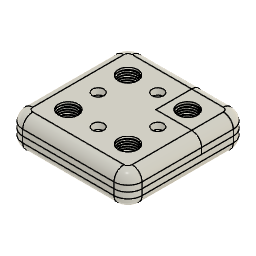
PTFE Mount (Autodesk Fusion 360 design; units mm, degrees)
Autodesk Fusion 360 part; units mm, degrees
sketch "Sketch1" plane through (0, 0, 0) normal (0, 0, 1) x (1, 0, 0)
  line L0 (-30, 0) -> (-30, 30)
  line L1 (-30, 30) -> (0, 30)
  line L2 (-30, 30) -> (30, 30)
  line L3 (30, 30) -> (30, -30)
  line L4 (30, -30) -> (-30, -30)
  line L5 (-30, -30) -> (-30, 30)
  line L6 (-20, 30) -> (-15, 30)
  line L7 (-30, 15) -> (-30, 20)
  point P0 (-15, 15)
  point P1 (15, 15)
  point P2 (15, -15)
  point P3 (-15, -15)
  point P4 (-30, 20)
  point P5 (-20, 30)
  dimension "d1" = 30
  dimension "d2" = 30
  dimension "d3" = 60
  dimension "d4" = 60
  constraint vertical L0
  constraint horizontal L1
  constraint horizontal L2
  constraint vertical L3
  constraint horizontal L4
  constraint vertical L5
  constraint horizontal L6
  constraint vertical L7
  constraint coincident P4 L7.end
  constraint coincident P5 L6.start
  measures "d1" distance of origin L0.start
  measures "d2" distance of origin L1.end
  measures "d3" distance of L0.end L2.end
  measures "d4" distance of L0.end L4.end
extrude "Extrude1" add sketch "Sketch1" along normal blind 8 makes body 1
sketch "Sketch2" plane through (0, 0, 8) normal (0, 0, 1) x (-1, 0, 0)
  line L0 (30, -30) -> (30, 30)
  line L1 (30, 30) -> (-30, 30)
  line L2 (-30, 30) -> (-30, -30)
  line L3 (-30, -30) -> (30, -30)
  circle A0 centre (15, -15) radius 2.075
  point P0 (15, -15)
cylinder "CylinderPrimitive1" cut diameter 4.25 height -14 placed x (1, 0, 0) y (0, 1, 0) z (0, 0, 1) at (-15, 15, 8) bodies 1
cylinder "CylinderPrimitive2" cut diameter 4.25 height -26 placed x (1, 0, 0) y (0, 1, 0) z (0, 0, 1) at (15, 15, 8) bodies 1
cylinder "CylinderPrimitive3" cut diameter 4.25 height -29 placed x (1, 0, 0) y (0, 1, 0) z (0, 0, 1) at (-15, -15, 8) bodies 1
cylinder "CylinderPrimitive4" cut diameter 4.25 height -23 placed x (1, 0, 0) y (0, 1, 0) z (0, 0, 1) at (15, -15, 8) bodies 1
sketch "Sketch10" plane through (0, 0, 8) normal (0, 0, 1) x (-1, 0, 0)
  point P0 (-15, -15)
  point P1 (-15, -15)
  point P2 (-15, 15)
  point P3 (-15, 15)
  point P4 (15, 15)
  point P5 (15, 15)
  constraint coincident P0 P1
  constraint coincident P2 P3
  constraint coincident P4 P5
hole "Hole1" at (-15, 15, 8) at (15, 15, 8) at (15, -15, 8) at (-15, -15, 8) direction (0, 0, -1) diameter 8.526 depth 6.5 tip angle 180 counterbore diameter 9.75 counterbore depth 1 bodies 1
thread "Thread1" "ISO Metric profile 10.0 M10x1.12 6H" major diameter 10.1608 minor diameter 8.9126 pitch 1.12 angle 60 modelled right hand crest width 0.306 on face at (-14.7875, 10.7423, 5.1667) crest through (-10.5437, 15, 6.72) on face at (15.2125, 10.7423, 5.1667) crest through (19.4563, 15, 6.72) on face at (15.2125, -19.2577, 5.1667) crest through (19.4563, -15, 6.72) on face at (-14.7875, -19.2577, 5.1667) crest through (-10.5437, -15, 6.72) on bodies 1
fillet "Fillet1" chord length 10 1 edges at (-30, -30, 4) on bodies 1
fillet "Fillet2" chord length 10 3 edges at (30, -30, 4) (30, 30, 4) (-30, 30, 4) on bodies 1
fillet "Fillet3" radius 5 8 edges at (27.9294, -27.9285, 8) (30, 0, 8) (27.9285, 27.9294, 8) (0, 30, 8) (-27.9294, 27.9285, 8) (-30, 0, 8) (-27.9285, -27.9294, 8) (0, -30, 8) on bodies 1
copy_body "CopyPasteBodies1" bodies 1 makes body 2
move_body "Move1" bodies 2 to x (-1, 0, 0) y (0, 1, 0) z (0, 0, -1) at (0, 0, 0)
sketch "Sketch11" plane through (0, 0, 8) normal (0, 0, 1) x (-1, 0, 0)
  circle A0 centre (15, 15) radius 4.875
  circle A1 centre (-15, -15) radius 4.875
  circle A2 centre (15, -15) radius 4.875
  circle A3 centre (-15, 15) radius 4.875
  spline S0 degree 3 poles (-25, 22.9289) (-25, 23.0652) (-24.9865, 23.2015) (-24.917, 23.549) (-24.8402, 23.756) (-24.5939, 24.1929) (-24.4033, 24.4108) (-23.9063, 24.7861) (-23.5846, 24.9225) (-23.1435, 24.9917) (-23.0362, 25) (-22.9289, 25) knots 0 0 0 0 0.040888 0.040888 0.106308 0.106308 0.191354 0.191354 0.293128 0.293128 0.325306 0.325306 0.325306 0.325306
  line L0 (-25, 22.9289) -> (-25, -22.9289)
  spline S1 degree 3 poles (-22.9289, -25) (-23.0652, -25) (-23.2015, -24.9865) (-23.549, -24.917) (-23.756, -24.8402) (-24.1929, -24.5939) (-24.4108, -24.4033) (-24.7861, -23.9063) (-24.9225, -23.5846) (-24.9917, -23.1435) (-25, -23.0362) (-25, -22.9289) knots 0 0 0 0 0.040888 0.040888 0.106308 0.106308 0.191354 0.191354 0.293128 0.293128 0.325306 0.325306 0.325306 0.325306
  line L1 (-22.9289, -25) -> (22.9289, -25)
  spline S2 degree 3 poles (25, -22.9289) (25, -23.0652) (24.9865, -23.2015) (24.917, -23.549) (24.8402, -23.756) (24.5939, -24.1929) (24.4033, -24.4108) (23.9063, -24.7861) (23.5846, -24.9225) (23.1435, -24.9917) (23.0362, -25) (22.9289, -25) knots 0 0 0 0 0.040888 0.040888 0.106308 0.106308 0.191354 0.191354 0.293128 0.293128 0.325306 0.325306 0.325306 0.325306
  line L2 (25, -22.9289) -> (25, 22.9289)
  spline S3 degree 3 poles (22.9289, 25) (23.0652, 25) (23.2015, 24.9865) (23.549, 24.917) (23.756, 24.8402) (24.1929, 24.5939) (24.4108, 24.4033) (24.7861, 23.9063) (24.9225, 23.5846) (24.9917, 23.1435) (25, 23.0362) (25, 22.9289) knots 0 0 0 0 0.040888 0.040888 0.106308 0.106308 0.191354 0.191354 0.293128 0.293128 0.325306 0.325306 0.325306 0.325306
  line L3 (22.9289, 25) -> (-22.9289, 25)
  point P0 (15, 0)
  point P1 (0, -15)
  point P2 (-15, 0)
  point P3 (0, 15)
  dimension "d31" = 15
  dimension "d32" = 15
  dimension "d33" = 15
  dimension "d34" = 15
  measures "d31" distance of origin P0
  measures "d32" distance of origin P2
  measures "d33" distance of origin P1
  measures "d34" distance of origin P3
hole "Hole2" at (0, 15, 8) at (-15, 0, 8) at (15, 0, 8) at (0, -15, 8) direction (0, 0, -1) diameter 3.2 depth 16 tip angle 180 counterbore diameter 5.75 counterbore depth 3.2 bodies 1
sketch "Sketch12" plane through (0, 0, -8) normal (0, 0, -1) x (1, 0, 0)
  circle A0 centre (15, 15) radius 4.875
  circle A1 centre (-15, -15) radius 4.875
  circle A2 centre (15, -15) radius 4.875
  circle A3 centre (-15, 15) radius 4.875
  spline S0 degree 3 poles (-25, 22.9289) (-25, 23.0652) (-24.9865, 23.2015) (-24.917, 23.549) (-24.8402, 23.756) (-24.5939, 24.1929) (-24.4033, 24.4108) (-23.9063, 24.7861) (-23.5846, 24.9225) (-23.1435, 24.9917) (-23.0362, 25) (-22.9289, 25) knots 0 0 0 0 0.040888 0.040888 0.106308 0.106308 0.191354 0.191354 0.293128 0.293128 0.325306 0.325306 0.325306 0.325306
  line L0 (-25, 22.9289) -> (-25, -22.9289)
  spline S1 degree 3 poles (-22.9289, -25) (-23.0652, -25) (-23.2015, -24.9865) (-23.549, -24.917) (-23.756, -24.8402) (-24.1929, -24.5939) (-24.4108, -24.4033) (-24.7861, -23.9063) (-24.9225, -23.5846) (-24.9917, -23.1435) (-25, -23.0362) (-25, -22.9289) knots 0 0 0 0 0.040888 0.040888 0.106308 0.106308 0.191354 0.191354 0.293128 0.293128 0.325306 0.325306 0.325306 0.325306
  line L1 (-22.9289, -25) -> (22.9289, -25)
  spline S2 degree 3 poles (25, -22.9289) (25, -23.0652) (24.9865, -23.2015) (24.917, -23.549) (24.8402, -23.756) (24.5939, -24.1929) (24.4033, -24.4108) (23.9063, -24.7861) (23.5846, -24.9225) (23.1435, -24.9917) (23.0362, -25) (22.9289, -25) knots 0 0 0 0 0.040888 0.040888 0.106308 0.106308 0.191354 0.191354 0.293128 0.293128 0.325306 0.325306 0.325306 0.325306
  line L2 (25, -22.9289) -> (25, 22.9289)
  spline S3 degree 3 poles (22.9289, 25) (23.0652, 25) (23.2015, 24.9865) (23.549, 24.917) (23.756, 24.8402) (24.1929, 24.5939) (24.4108, 24.4033) (24.7861, 23.9063) (24.9225, 23.5846) (24.9917, 23.1435) (25, 23.0362) (25, 22.9289) knots 0 0 0 0 0.040888 0.040888 0.106308 0.106308 0.191354 0.191354 0.293128 0.293128 0.325306 0.325306 0.325306 0.325306
  line L3 (22.9289, 25) -> (-22.9289, 25)
  line L4 (-17.9055, 1.6058) -> (-17.8435, -1.7134)
  line L5 (-17.8435, -1.7134) -> (-14.9379, -3.3192)
  line L6 (-14.9379, -3.3192) -> (-12.0945, -1.6058)
  line L7 (-12.0945, -1.6058) -> (-12.1565, 1.7134)
  line L8 (-12.1565, 1.7134) -> (-15.0621, 3.3192)
  line L9 (-15.0621, 3.3192) -> (-17.9055, 1.6058)
  line L10 (12.1483, 1.6996) -> (12.1023, -1.6199)
  line L11 (12.1023, -1.6199) -> (14.954, -3.3194)
  line L12 (14.954, -3.3194) -> (17.8517, -1.6996)
  line L13 (17.8517, -1.6996) -> (17.8977, 1.6199)
  line L14 (17.8977, 1.6199) -> (15.046, 3.3194)
  line L15 (15.046, 3.3194) -> (12.1483, 1.6996)
  line L16 (-1.6599, 17.875) -> (-3.3198, 15)
  line L17 (-3.3198, 15) -> (-1.6599, 12.125)
  line L18 (-1.6599, 12.125) -> (1.6599, 12.125)
  line L19 (1.6599, 12.125) -> (3.3198, 15)
  line L20 (3.3198, 15) -> (1.6599, 17.875)
  line L21 (1.6599, 17.875) -> (-1.6599, 17.875)
  line L22 (-1.6599, -12.125) -> (-3.3198, -15)
  line L23 (-3.3198, -15) -> (-1.6599, -17.875)
  line L24 (-1.6599, -17.875) -> (1.6599, -17.875)
  line L25 (1.6599, -17.875) -> (3.3198, -15)
  line L26 (3.3198, -15) -> (1.6599, -12.125)
  line L27 (1.6599, -12.125) -> (-1.6599, -12.125)
  point P0 (0, -15)
  point P1 (0, -15)
  point P2 (-15, 0)
  point P3 (-15, 0)
  point P4 (0, 15)
  point P5 (0, 15)
  point P6 (15, 0)
  point P7 (15, 0)
  point P8 (-15, 0)
  point P9 (15, 0)
  point P10 (0, 15)
  point P11 (0, -15)
  dimension "d40" = 2.875
  dimension "d41" = 2.875
  dimension "d42" = 2.875
  dimension "d43" = 2.875
  constraint coincident P11 P1
  constraint coincident P8 P3
  constraint coincident P10 P5
  constraint coincident P9 P7
  measures "d40" distance of P8 L9
  measures "d41" distance of P9 L15
  measures "d42" distance of P10 L21
  measures "d43" distance of P11 L27
extrude "Extrude2" cut sketch "Sketch12" against normal blind 4.7 contours L4 L5 L6 L7 L8 L9 | L10 L11 L12 L13 L14 L15 | L16 L17 L18 L19 L20 L21 | L22 L23 L24 L25 L26 L27 bodies 2
sketch "Sketch13" plane through (0, 0, -8) normal (0, 0, -1) x (1, 0, 0)
  point P0 (-15, 15)
  point P1 (-15, 15)
  point P2 (15, 15)
  point P3 (15, 15)
  point P4 (15, -15)
  point P5 (15, -15)
  point P6 (-15, -15)
  point P7 (-15, -15)
  point P8 (0, 15)
  point P9 (0, 15)
  point P10 (-15, 0)
  point P11 (-15, 0)
  point P12 (15, 0)
  point P13 (15, 0)
  point P14 (0, -15)
  point P15 (0, -15)
  constraint coincident P0 P1
  constraint coincident P2 P3
  constraint coincident P4 P5
  constraint coincident P6 P7
  constraint coincident P8 P9
  constraint coincident P10 P11
  constraint coincident P12 P13
  constraint coincident P14 P15
hole "Hole3" at (0, -15, -8) at (15, 0, -8) at (0, 15, -8) at (-15, 0, -8) direction (0, 0, 1) diameter 3.2 depth 16 tip angle 180 bodies 2
copy_body "Body->Comp1" bodies 2 removing the originals makes body 3 in component "PTFE Mount Rear"
copy_body "Body->Comp2" bodies 1 removing the originals makes body 4 in component "PTFE Mount Front"
copy_body "CopyPasteBodies2" bodies 4 makes body 5
ref_plane "WorkPlane1" through (7, 0, 1.5) normal (1, 0, 0) x (0, 1, 0)
ref_plane "WorkPlane2" through (0, 7, 1.5) normal (0, 1, 0) x (-1, 0, 0)
split "Split1" by plane through (7, 0, 1.5) normal (1, 0, 0) bodies 5 makes body 6 at (25.5318, 0.0399, 0)
split "Split2" by plane through (0, 7, 1.5) normal (0, 1, 0) bodies 6 makes body 7 at (14.9234, 25.7064, 0)
delete_body "RemoveBody3" bodies 5
delete_body "RemoveBody4" bodies 6
component "PTFE Mount Rear" placed x (1, 0, 0) y (0, 1, 0) z (0, 0, 1) at (0, 0, 0)
component "PTFE Mount Front" placed x (1, 0, 0) y (0, 1, 0) z (0, 0, 1) at (0, 0, 0)
